upper stabeliser (Autodesk Fusion 360 design; units mm, degrees)
Autodesk Fusion 360 part; units mm, degrees
sketch "Sketch1" plane through (0, 0, 28.25) normal (0, 0, 1) x (-1, 0, 0)
  circle A0 centre (0, -20.5) radius 4.05
  arc A1 (7.8309, -11.66) -> (11.4059, -8.085) centre (7.8309, -8.085) ccw
  line L0 (7.8309, -11.66) -> (-8.1691, -11.66)
  arc A2 (-11.7441, -8.0962) -> (-8.1691, -11.66) centre (-8.1691, -8.085) ccw
  line L1 (-11.7441, -8.0962) -> (-11.7941, 7.9538)
  arc A3 (-8.2191, 11.54) -> (-11.7941, 7.9538) centre (-8.2191, 7.965) ccw
  line L2 (-8.2191, 11.54) -> (7.8309, 11.54)
  arc A4 (11.4059, 7.965) -> (7.8309, 11.54) centre (7.8309, 7.965) ccw
  line L3 (11.4059, 7.965) -> (11.4059, -8.085)
  line L4 (-12.5, 14.5) -> (-12.5, -5.6)
  line L5 (-12.5, -5.6) -> (-26, -5.6)
  line L6 (-26, -5.6) -> (-26, -15.5)
  line L7 (-26, -15.5) -> (-12.5, -15.5)
  line L8 (-12.5, -15.5) -> (-12.5, -26.5)
  line L9 (-12.5, -26.5) -> (12.5, -26.5)
  line L10 (12.5, -26.5) -> (12.5, -15.5)
  line L11 (12.5, -15.5) -> (26, -15.5)
  line L12 (26, -15.5) -> (26, -5.6)
  line L13 (26, -5.6) -> (12.5, -5.6)
  line L14 (12.5, -5.6) -> (12.5, 14.5)
  line L15 (12.5, 14.5) -> (-12.5, 14.5)
  circle A5 centre (0, -20.5) radius 4.05
  circle A6 centre (0, -20.5) radius 6
  circle A7 centre (0, -60.5) radius 1.25
  circle A8 centre (0, -60.5) radius 5
  line L16 (5, -60.5) -> (-5, -60.5) construction
  line L17 (-5, -60.5) -> (-5, -20.5)
  line L18 (-5, -20.5) -> (5, -20.5) construction
  line L19 (5, -20.5) -> (5, -60.5)
  dimension "d144" = 8.1
  dimension "d145" = 12
  dimension "d146" = 10
  dimension "d1" = 40
  constraint concentric A0 A5
  constraint concentric A5 A6
  constraint concentric A7 A8
  constraint horizontal L16
  constraint vertical L17
  constraint horizontal L18
  constraint vertical L19
  constraint midpoint A0.centre L18
  constraint midpoint A7.centre L16
  constraint coincident A8 L16.start
  measures "d144" diameter of A5
  measures "d145" diameter of A6
  measures "d146" diameter of A8
  measures "d1" distance of L16.end L17.end
extrude "Extrude1" add sketch "Sketch1" along normal blind 4 contours L9 A6 L17 | L9 A8 L17 L19 | L9 A6 L19 | A6 | A8 | A7
sketch "Sketch2" plane through (0, 0, 28.25) normal (0, 0, -1) x (1, 0, 0)
  circle A0 centre (0, -20.5) radius 4.05
  arc A1 (-5, -60.5) -> (5, -60.5) centre (0, -60.5) ccw
  line L0 (5, -60.5) -> (5, -23.8166)
  arc A2 (5, -23.8166) -> (-5, -23.8166) centre (0, -20.5) ccw
  line L1 (-5, -23.8166) -> (-5, -60.5)
  circle A3 centre (0, -60.5) radius 2.95
  dimension "d149" = 5.9
  constraint concentric A1 A3
  measures "d149" diameter of A3
extrude "Extrude2" add sketch "Sketch2" along normal blind 7.5 contours A3
sketch "Sketch3" plane through (0, 0, 32.25) normal (0, 0, 1) x (-1, 0, 0)
  circle A0 centre (0, -20.5) radius 4.05
  arc A1 (-5, -60.5) -> (5, -60.5) centre (0, -60.5) ccw
  line L0 (5, -60.5) -> (5, -23.8166)
  arc A2 (5, -23.8166) -> (-5, -23.8166) centre (0, -20.5) ccw
  line L1 (-5, -23.8166) -> (-5, -60.5)
  circle A3 centre (0, -60.5) radius 0.8
  dimension "d152" = 1.6
  constraint concentric A1 A3
  measures "d152" diameter of A3
extrude "Extrude3" cut sketch "Sketch3" against normal blind 14 contours A3
